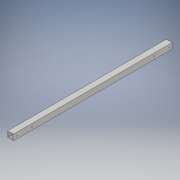
# Autodesk Inventor part: 1x1 27 362in
Saved by Autodesk Inventor 2018 (Build 220112000, 112)
## iProperties
Created: 2019-01-19
Part Number: 1x1 27 362in
Material: Generic
Document SubType Name: Modeling
Designer: maste
Density: 1 g/cm^3
Appearance: Default
Author: maste
Autodesk Inventor part; units mm, degrees
ref_plane "YZ Plane" through (0, 0, 0) normal (1, 0, 0) x (0, 1, 0)
ref_plane "XZ Plane" through (0, 0, 0) normal (0, 1, 0) x (-1, 0, 0)
ref_plane "XY Plane" through (0, 0, 0) normal (0, 0, 1) x (1, 0, 0)
sketch "Sketch1" plane through (0, 0, 0) normal (0, 0, 1) x (1, 0, 0)
  line L0 (0, 0) -> (25.4, 0)
  line L1 (25.4, 0) -> (25.4, 25.4)
  line L2 (25.4, 25.4) -> (0, 25.4)
  line L3 (0, 25.4) -> (0, 0)
  line L4 (3.175, 3.175) -> (22.225, 3.175)
  line L5 (22.225, 3.175) -> (22.225, 22.225)
  line L6 (22.225, 22.225) -> (3.175, 22.225)
  line L7 (3.175, 22.225) -> (3.175, 3.175)
  dimension "d0" = 25.4
  dimension "d1" = 25.4
  dimension "d2" = 3.175
  constraints: 16 end point, 4 parallel, 2 perpendicular, 1 horizontal, 3 other
  measures "d0" distance of L2.end L1.end
  measures "d1" distance of L1.end L0.end
  measures "d2" distance between parallel lines of L3 L7
extrude "Extrusion1" add sketch "Sketch1" along normal blind 694.9948
sketch "Sketch2" plane through (25.4, 0, 0) normal (1, 0, 0) x (0, 0, -1)
  line L0 (0, 3.175) -> (0, 22.225) construction
  line L1 (0, 12.7) -> (-12.7, 12.7) construction
  line L2 (-694.9948, 22.225) -> (-694.9948, 3.175) construction
  line L3 (-694.9948, 12.7) -> (-682.2948, 12.7) construction
  circle A0 centre (-682.2948, 12.7) radius 2.5019
  circle A1 centre (-12.7, 12.7) radius 2.5019
  line L4 (-682.2948, 12.7) -> (-615.442, 12.7) construction
  line L5 (-12.7, 12.7) -> (-79.5528, 12.7) construction
  circle A2 centre (-79.5528, 12.7) radius 2.5019
  circle A3 centre (-615.442, 12.7) radius 2.5019
  point P0 (0, 0)
  dimension "d5" = 12.7
  dimension "d7" = 12.7
  dimension "d8" = 5.0038
  dimension "d11" = 66.8528
  dimension "d12" = 66.8528
  constraints: 8 end point, 4 centre point, 4 coincident, 4 horizontal, 2 midpoint
  measures "d5" distance of L1.start L1.end
  measures "d7" distance of L3.start L3.end
  measures "d8" diameter of A0
  measures "d11" distance of L4.start L4.end
  measures "d12" distance of L5.start L5.end
extrude "Extrusion3" cut sketch "Sketch2" against normal blind 694.9948
body "Solid1"
